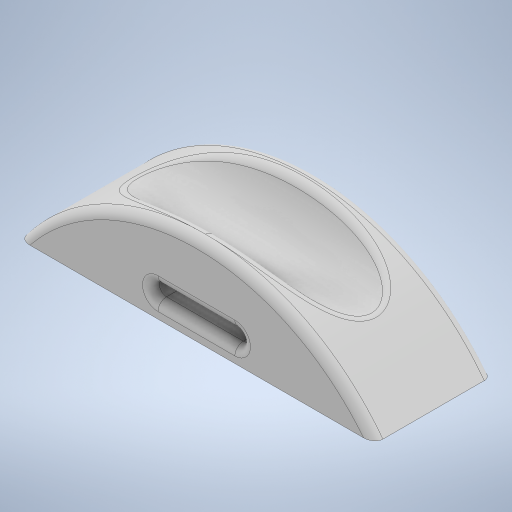
# Autodesk Inventor part: cuff
Saved by Autodesk Inventor 2024 (Build 280153000, 153)
## iProperties
Created: 2023-09-09
Part Number: cuff
Material: Generic
Document SubType Name: Modeling
Designer: Pintu
Density: 1 g/cm^3
Appearance: Default
Author: Pintu
Autodesk Inventor part; units mm, degrees
ref_plane "YZ Plane" through (0, 0, 0) normal (1, 0, 0) x (0, 1, 0)
ref_plane "XZ Plane" through (0, 0, 0) normal (0, 1, 0) x (-1, 0, 0)
ref_plane "XY Plane" through (0, 0, 0) normal (0, 0, 1) x (1, 0, 0)
sketch "Sketch1" plane through (0, 0, 0) normal (0, 0, 1) x (1, 0, 0)
  arc A0 (120, 0) -> (-120, 0) centre (0, -90) ccw
  line L0 (-120, 0) -> (120, 0)
  point P0 (0, 0)
  dimension "d0" = 240
  dimension "d1" = 150
  dimension "d2" = 120
  constraints: 2 end point, 2 horizontal alignment, 2 point on circle, 1 centre point, 1 horizontal
  measures "d0" distance of L0.start L0.end
  measures "d1" radius of A0
  measures "d2" distance of L0.start point (0, 0)
extrude "Extrusion1" add sketch "Sketch1" along normal mid plane 80
sketch "Sketch2" plane through (0, 0, 0) normal (1, 0, 0) x (0, 1, 0)
  line L0 (60, -40) -> (60, 40) projected
  arc A0 (60, 30) -> (60, -28.5626) centre (66.5274, 0.7187) ccw
  point P0 (0, 0)
  point P1 (60, 0)
  dimension "d5" = 30
  dimension "d6" = 30
  constraints: 2 point on circle, 2 point on line, 1 centre point, 1 midpoint
  measures "d5" radius of A0
  measures "d6" distance of point (60, 0) A0.start
extrude "Extrusion2" cut sketch "Sketch2" along normal mid plane 500
fillet "Fillet1" radius 5.75 4 edges at (-80.565, 36.5278, 0.8767) (80.565, 36.5278, 0.8767) (0, 60, 40) (0, 60, -40)
sketch "Sketch3" plane through (0, 0, 40) normal (0, 0, 1) x (1, 0, 0)
  line L0 (-26.2135, 14.9328) -> (25.7266, 14.9328) construction
  line L1 (-26.2135, 10.2006) -> (25.7266, 10.2006)
  line L2 (25.7266, 19.665) -> (-26.2135, 19.665)
  arc A0 (-26.2135, 19.665) -> (-26.2135, 10.2006) centre (-26.2135, 14.9328) ccw
  arc A1 (25.7266, 10.2006) -> (25.7266, 19.665) centre (25.7266, 14.9328) ccw
  point P0 (0, 0)
  point P1 (-0.2435, 14.9328)
  constraints: 8 end point, 4 point on circle, 4 tangent, 2 centre point, 1 horizontal, 1 midpoint, 1 parallel
extrude "Extrusion3" cut sketch "Sketch3" against normal blind 500
fillet "Fillet2" radius 5.75 8 edges at (30.4588, 14.9328, 40) (-0.2435, 10.2006, 40) (-30.9457, 14.9328, 40) (-0.2435, 19.665, 40) (30.4588, 14.9328, -40) (-0.2435, 19.665, -40) (-30.9457, 14.9328, -40) (-0.2435, 10.2006, -40)
body "Solid1"
